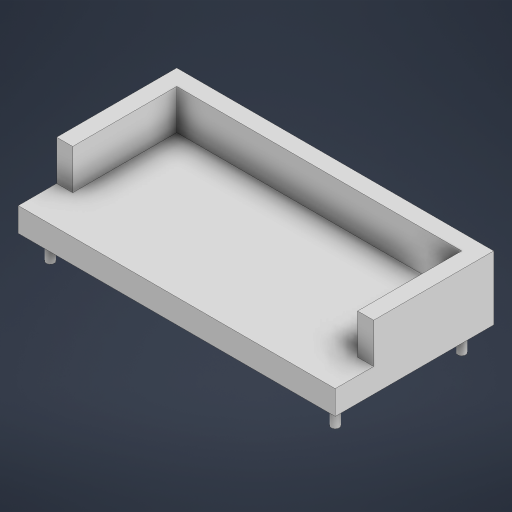
# Autodesk Inventor part: Divano
Saved by Autodesk Inventor 2024.2 (Build 282272000, 272)
## iProperties
Created: 2025-08-11
Part Number: Divano
Material: Generic
Document SubType Name: Modeling
Designer: Luca
Density: 1 g/cm^3
Appearance: Default
Author: Luca
Autodesk Inventor part; units mm, degrees
ref_plane "YZ Plane" through (0, 0, 0) normal (1, 0, 0) x (0, 1, 0)
ref_plane "XZ Plane" through (0, 0, 0) normal (0, 1, 0) x (-1, 0, 0)
ref_plane "XY Plane" through (0, 0, 0) normal (0, 0, 1) x (1, 0, 0)
sketch "Sketch1" plane through (0, 0, 0) normal (0, 1, 0) x (-1, 0, 0)
  line L0 (990, 495) -> (-990, 495) construction
  line L1 (-990, 495) -> (-990, -495) construction
  line L2 (-990, -495) -> (990, -495) construction
  line L3 (990, -495) -> (990, 495) construction
  line L4 (990, 495) -> (-990, -495) construction
  line L5 (-990, 495) -> (990, -495) construction
  line L6 (890, -395) -> (-890, -395) construction
  line L7 (-890, -395) -> (-890, 395) construction
  line L8 (-890, 395) -> (890, 395) construction
  line L9 (890, 395) -> (890, -395) construction
  circle A0 centre (890, -395) radius 25
  circle A1 centre (-890, -395) radius 25
  circle A2 centre (890, 395) radius 25
  circle A3 centre (-890, 395) radius 25
  point P0 (0, 0)
  dimension "d0" = 1980
  dimension "d1" = 990
  dimension "d2" = 100
  dimension "d3" = 50
  constraints: 20 end point, 4 centre point, 4 coincident, 4 parallel, 3 equal radius, 2 midpoint, 2 perpendicular, 1 horizontal, 3 other
  measures "d0" distance of L2.end L1.end
  measures "d1" distance of L1.end L0.end
  measures "d2" distance between parallel lines of L2 L6
  measures "d3" diameter of A0
extrude "Extrusion1" add sketch "Sketch1" along normal blind 150
sketch "Sketch2" plane through (0, 150, 0) normal (0, 1, 0) x (-1, 0, 0)
  line L0 (990, -495) -> (990, 495) projected
  line L1 (-990, -495) -> (990, -495) projected
  line L2 (-990, 495) -> (-990, -495) projected
  line L3 (990, 495) -> (-990, 495) projected
  point P0 (0, 0)
extrude "Extrusion2" add sketch "Sketch2" along normal blind 150
sketch "Sketch3" plane through (0, 300, 0) normal (0, 1, 0) x (1, 0, 0)
  line L0 (-990, 495) -> (990, 495)
  line L1 (990, 495) -> (990, 395)
  line L2 (990, 395) -> (-990, 395)
  line L3 (-990, 395) -> (-990, 495)
  line L4 (990, 395) -> (890, 395)
  line L5 (890, 395) -> (890, -255)
  line L6 (890, -255) -> (990, -255)
  line L7 (990, -255) -> (990, 395)
  line L8 (-990, 395) -> (-890, 395)
  line L9 (-890, 395) -> (-890, -255)
  line L10 (-890, -255) -> (-990, -255)
  line L11 (-990, -255) -> (-990, 395)
  line L12 (990, -495) -> (990, 495) projected
  point P0 (0, 0)
  dimension "d8" = 100
  dimension "d10" = 650
  constraints: 24 end point, 6 parallel, 3 horizontal, 3 perpendicular, 2 equal length, 1 collinear, 1 point on line
  measures "d8" distance of L0.end L1.end
  measures "d10" distance of L5.end L4.end
extrude "Extrusion3" add sketch "Sketch3" along normal blind 250
body "Solid1"
